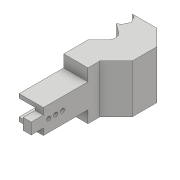
# Autodesk Inventor part: rec_c_16mm_x_60mm
Saved by Autodesk Inventor 2017 (Build 210142000, 142)
## iProperties
Created: 2018-04-21
Part Number: rec_c_16mm_x_60mm
Material: Generic
Document SubType Name: Modeling
Designer: Jeyy
Density: 1 g/cm^3
Appearance: Default
Author: Jeyy
Autodesk Inventor part; units mm, degrees
ref_plane "YZ Plane" through (0, 0, 0) normal (1, 0, 0) x (0, 1, 0)
ref_plane "XZ Plane" through (0, 0, 0) normal (0, 1, 0) x (-1, 0, 0)
sketch "Sketch1" plane through (0, 0, 0) normal (0, 0, 1) x (1, 0, 0)
  line L0 (0, 0) -> (25, 0)
  line L1 (25, 0) -> (25, 40)
  line L2 (25, 40) -> (0, 40)
  line L3 (0, 40) -> (0, 0)
  dimension "d1" = 25
  dimension "d2" = 40
  dimension "d3" = 25
  constraints: 8 end point, 2 perpendicular, 1 horizontal
  measures "d1" distance of L0.start L0.end
  measures "d2" distance of L0.end L1.end
  measures "d3" distance of L1.end L2.end
extrude "Extrusion1" add sketch "Sketch1" against normal blind 30
sketch "Sketch2" plane through (25, 0, 0) normal (1, 0, 0) x (0, 0, -1)
  line L0 (0, 0) -> (30, 0) projected
  circle A0 centre (15, 6.56) radius 2.46
  constraints: 1 centre point
extrude "Extrusion2" cut sketch "Sketch2" against normal blind 30
sketch "Sketch3" plane through (0, 0, 0) normal (-1, 0, 0) x (0, 0, 1)
  line L0 (0, 0) -> (-30, 0) projected
  line L1 (-25.05, 0) -> (-4.95, 0)
  line L2 (-4.95, 0) -> (-4.95, 33.12)
  line L3 (-4.95, 33.12) -> (-25.05, 33.12)
  line L4 (-25.05, 33.12) -> (-25.05, 0)
  dimension "d11" = 20.1
  constraints: 8 end point, 2 parallel, 1 perpendicular
  measures "d11" distance of L1.start L1.end
extrude "Extrusion3" cut sketch "Sketch3" against normal blind 20
sketch "Sketch4" plane through (0, 0, 0) normal (0, -1, 0) x (1, 0, 0)
  line L0 (20, -4.95) -> (20, -25.05) projected
  line L1 (20, -15) -> (25, -15)
  line L2 (25, 0) -> (25, -30) projected
  line L3 (20, -8.025) -> (25, -8.025)
  line L4 (25, -8.025) -> (25, -21.975)
  line L5 (25, -21.975) -> (20, -21.975)
  line L6 (20, -21.975) -> (20, -8.025)
  line L7 (20, -8.025) -> (25, -21.975) construction
  line L8 (25, -8.025) -> (20, -21.975) construction
  line L9 (25, -12.54) -> (25, -17.46) projected
  point P0 (0, 0)
  point P1 (22.5, -15)
  dimension "d14" = 13.95
  constraints: 14 end point, 5 midpoint, 2 parallel, 2 perpendicular
  measures "d14" distance of L3.end L4.end
extrude "Extrusion4" add sketch "Sketch4" along normal blind 15
sketch "Sketch5" plane through (20, 0, 0) normal (-1, 0, 0) x (0, 0, 1)
  circle A0 centre (-15, 6.56) radius 2.46 projected
  circle A1 centre (-15, 6.56) radius 4.7025
  circle A2 centre (-15, 6.56) radius 2.46 projected
  circle A3 centre (-15, 6.56) radius 2.46
  point P0 (0, 0)
  dimension "d17" = 9.405
  constraints: 2 centre point, 2 coincident
  measures "d17" diameter of A1
extrude "Extrusion5" cut sketch "Sketch5" against normal blind 2.1
sketch "Sketch6" plane through (25, 0, 0) normal (1, 0, 0) x (0, 0, -1)
  circle A0 centre (15, 6.56) radius 4.7025 projected
  line L0 (15, 6.56) -> (15, 23.56)
  circle A1 centre (15, 23.56) radius 2.46
  point P0 (0, 0)
  dimension "d20" = 17
  dimension "d21" = 4.92
  constraints: 2 end point, 1 centre point, 1 coincident, 1 vertical
  measures "d20" distance of L0.start L0.end
  measures "d21" diameter of A1
extrude "Extrusion6" cut sketch "Sketch6" against normal blind 10 contours A1
sketch "Sketch7" plane through (20, 0, 0) normal (-1, 0, 0) x (0, 0, 1)
  circle A0 centre (-15, 23.56) radius 2.46 projected
  circle A1 centre (-15, 23.56) radius 4.7025
  point P0 (0, 0)
  dimension "d24" = 9.405
  constraints: 1 centre point, 1 coincident
  measures "d24" diameter of A1
extrude "Extrusion7" cut sketch "Sketch7" against normal blind 2.1
sketch "Sketch9" plane through (25, 0, 0) normal (1, 0, 0) x (0, 0, -1)
  circle A0 centre (15, 6.56) radius 2.46 projected
  circle A1 centre (15, 6.56) radius 2.46
  circle A2 centre (15, 23.56) radius 2.46 projected
  circle A3 centre (15, 23.56) radius 2.46
  line L0 (30, 40) -> (30, 0) projected
  line L1 (30, 0) -> (30, 40)
  line L2 (30, 40) -> (0, 40)
  line L3 (0, 40) -> (0, 0)
  line L4 (0, 0) -> (8.025, 0) projected
  line L5 (21.975, 0) -> (21.975, -15)
  line L6 (21.975, -15) -> (8.025, -15)
  line L7 (8.025, -15) -> (8.025, 0)
  line L8 (0, 0) -> (8.025, 0)
  line L9 (21.975, 0) -> (30, 0)
  constraints: 16 end point, 4 parallel, 2 centre point, 2 coincident, 2 horizontal, 2 perpendicular
extrude "Extrusion8" add sketch "Sketch9" along normal blind 5
sketch "Sketch10" plane through (0, 40, 0) normal (0, 1, 0) x (1, 0, 0)
  line L0 (0, 30) -> (30, 30) projected
  line L1 (30, 0) -> (0, 0) projected
  line L2 (0, 30) -> (30, 30)
  line L3 (30, 30) -> (30, 0)
  line L4 (30, 0) -> (0, 0)
  line L5 (0, 0) -> (0, 30)
  constraints: 8 end point, 2 parallel, 1 horizontal, 1 perpendicular
extrude "Extrusion9" add sketch "Sketch10" along normal blind 30
sketch "Sketch12" plane through (30, 0, 0) normal (1, 0, 0) x (0, 0, -1)
  circle A0 centre (15, 6.56) radius 2.46 projected
  line L0 (15, 6.56) -> (15, 15.06)
  circle A1 centre (15, 15.06) radius 2.525
  point P0 (0, 0)
  dimension "d31" = 8.5
  dimension "d33" = 5.05
  constraints: 2 end point, 1 centre point, 1 coincident, 1 vertical
  measures "d31" distance of L0.start L0.end
  measures "d33" diameter of A1
extrude "Extrusion10" cut sketch "Sketch12" against normal blind 30 contours A1
sketch "Sketch15" plane through (0, 0, -25.05) normal (-1, 0, 0) x (0, 0, 1)
  line L0 (0, 33.12) -> (20.1, 33.12) projected
  line L1 (20.1, 33.12) -> (20.1, 0) projected
  line L2 (0, 33.12) -> (20.1, 33.12)
  line L3 (20.1, 33.12) -> (20.1, 31.1)
  line L4 (20.1, 31.1) -> (0, 31.1)
  line L5 (0, 31.1) -> (0, 33.12)
  point P0 (25.05, 0)
  dimension "d57" = 2.02
  constraints: 8 end point, 2 parallel, 1 horizontal, 1 perpendicular, 1 point on line
  measures "d57" distance of L2.end L3.end
extrude "Extrusion13" add sketch "Sketch15" against normal blind 20
sketch "Sketch17" plane through (0, 0, 0) normal (0, 0, 1) x (1, 0, 0)
  line L0 (0, 70) -> (30, 70) projected
  line L1 (30, 70) -> (50.0622, 90.0622)
  line L2 (30, 70) -> (80, 70) construction
  line L3 (11.9522, 97.2454) -> (0, 85.2932)
  line L4 (0, 70) -> (0, 85.2932)
  line L5 (0, 70) -> (0, 0) projected
  line L6 (0, 70) -> (30, 70)
  line L7 (10.923, 112.2849) -> (0, 120.567)
  line L8 (50.0622, 105.3553) -> (50.0622, 120.567)
  line L9 (50.0622, 105.3553) -> (50.0622, 90.0622)
  arc A0 (11.9522, 97.2454) -> (10.923, 112.2849) centre (4.8811, 104.3165) ccw
  line L10 (4, 138.567) -> (0, 140.567)
  line L11 (4, 122.567) -> (0, 120.567)
  line L12 (4, 122.567) -> (8, 130.567)
  line L13 (4, 138.567) -> (8, 130.567)
  line L14 (0, 140.567) -> (30, 140.567)
  line L15 (30, 140.567) -> (50.0622, 120.567)
  dimension "d61" = 45
  dimension "d62" = 32.0271
  dimension "d72" = 10
  constraints: 28 end point, 3 vertical, 2 point on circle, 2 tangent, 1 centre point, 1 collinear, 1 horizontal, 1 perpendicular
  measures "d61" angle of L2 L1
  measures "d62" distance between parallel lines of L1 L3
  measures "d72" radius of A0
extrude "Extrusion14" add sketch "Sketch17" against normal blind 30
sketch "Sketch21" plane through (0, 0, 0) normal (0, 0, 1) x (1, 0, 0)
  line L0 (50.0622, 90.0622) -> (30, 70) projected
  line L1 (30, 70) -> (50.0622, 90.0622)
  line L2 (50.0622, 90.0622) -> (50.0622, 120.567) projected
  line L3 (50.0622, 90.0622) -> (50.0622, 120.567)
  line L4 (0, 140.567) -> (30, 140.567) projected
  line L5 (50.0622, 120.567) -> (30, 140.567)
  line L6 (30, 140.567) -> (0, 140.567)
  line L7 (4, 138.567) -> (0, 140.567) projected
  line L8 (0, 140.567) -> (4, 138.567)
  line L9 (8, 130.567) -> (4, 138.567) projected
  line L10 (4, 138.567) -> (8, 130.567)
  line L11 (4, 122.567) -> (8, 130.567) projected
  line L12 (8, 130.567) -> (4, 122.567)
  line L13 (0, 120.567) -> (4, 122.567) projected
  line L14 (4, 122.567) -> (0, 120.567)
  line L15 (10.923, 112.2849) -> (0, 120.567) projected
  line L16 (0, 120.567) -> (10.923, 112.2849)
  line L17 (0, 85.2932) -> (11.9522, 97.2454) projected
  line L18 (11.9522, 97.2454) -> (0, 85.2932)
  line L19 (0, 85.2932) -> (0, 55.2932)
  line L20 (0, 55.2932) -> (30, 55.2932)
  line L21 (30, 55.2932) -> (30, 70)
  arc A0 (11.9522, 97.2454) -> (10.923, 112.2849) centre (4.8811, 104.3165) ccw
  dimension "d79" = 30
  dimension "d81" = 30
  constraints: 26 end point, 8 collinear, 2 point on circle, 1 centre point, 1 horizontal, 1 perpendicular, 1 tangent
  measures "d79" distance of L17.start L19.end
  measures "d81" distance of L19.end L20.end
extrude "Extrusion15" add sketch "Sketch21" along normal blind 15
ref_plane "Work Plane1" through (0, 0, -15) normal (0, 0, 1) x (1, 0, 0)
mirror "Mirror1" about plane through (0, 0, -15) normal (0, 0, 1) of "Extrusion15"
body "Solid1"
